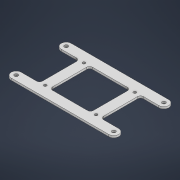
# Autodesk Inventor part: Mount Base
Saved by Autodesk Inventor 2021 (Build 250183000, 183)
## iProperties
Created: 2025-01-15
Part Number: Mount Base
Material: Generic
Document SubType Name: Modeling
Designer: user
Density: 1 g/cm^3
Appearance: Default
Author: user
Autodesk Inventor part; units mm, degrees
ref_plane "YZ Plane" through (0, 0, 0) normal (1, 0, 0) x (0, 1, 0)
ref_plane "XZ Plane" through (0, 0, 0) normal (0, 1, 0) x (-1, 0, 0)
ref_plane "XY Plane" through (0, 0, 0) normal (0, 0, 1) x (1, 0, 0)
sketch "Sketch1" plane through (0, 0, 0) normal (0, 1, 0) x (-1, 0, 0)
  line L0 (-7, 37.9777) -> (-7, 79.4722)
  spline S0 degree 3 poles (-7, 79.4722) (-7, 80.2679) (-6.8804, 81.313) (-5.8043, 84.1015) (-4.8936, 85.3942) (-3.1709, 87.6073) (-2.4028, 88.4658) (-2.0131, 89.2627) (-1.9647, 89.4035) (-1.9309, 89.6007) (-1.9254, 89.6626) (-1.9254, 89.7249) knots 0 0 0 0 0.238712 0.238712 0.524177 0.524177 0.81278 0.81278 0.88277 0.88277 0.915008 0.915008 0.915008 0.915008
  line L1 (0, 89.7249) -> (-1.9254, 89.7249)
  line L2 (0, 111.4478) -> (0, 89.7249)
  arc A0 (-6.2149, 117.4498) -> (0, 111.4478) centre (-2.5273, 115.0495) ccw
  line L3 (-135.9053, 117.4498) -> (-6.2149, 117.4498)
  arc A1 (-141.8339, 111.5213) -> (-135.9053, 117.4498) centre (-139.8146, 115.4305) ccw
  line L4 (-141.8339, 89.7249) -> (-141.8339, 111.5213)
  line L5 (-139.9085, 89.7249) -> (-141.8339, 89.7249)
  spline S1 degree 3 poles (-134.8339, 79.4722) (-134.8339, 80.1182) (-134.9165, 80.7597) (-135.2383, 82.0916) (-135.4922, 82.7684) (-136.3337, 84.5039) (-137.0038, 85.4638) (-138.2583, 87.0963) (-138.8405, 87.7821) (-139.5233, 88.7046) (-139.7055, 88.9932) (-139.8538, 89.363) (-139.888, 89.4816) (-139.9062, 89.645) (-139.9085, 89.685) (-139.9085, 89.7249) knots -1.843204 -1.843204 -1.843204 -1.843204 -1.717345 -1.717345 -1.576636 -1.576636 -1.342905 -1.342905 -1.132569 -1.132569 -0.995579 -0.995579 -0.934295 -0.934295 -0.914246 -0.914246 -0.914246 -0.914246
  line L6 (-134.8339, 79.4722) -> (-134.8339, 37.9777)
  spline S2 degree 3 poles (-134.8339, 37.9777) (-134.8339, 37.182) (-134.9535, 36.1368) (-136.0296, 33.3484) (-136.9403, 32.0557) (-138.663, 29.8425) (-139.4311, 28.984) (-139.8208, 28.1872) (-139.8692, 28.0464) (-139.903, 27.8492) (-139.9085, 27.7873) (-139.9085, 27.7249) knots 0 0 0 0 0.238712 0.238712 0.524177 0.524177 0.81278 0.81278 0.88277 0.88277 0.915008 0.915008 0.915008 0.915008
  line L7 (-141.8339, 27.7249) -> (-139.9085, 27.7249)
  line L8 (-141.8339, 5.9286) -> (-141.8339, 27.7249)
  arc A2 (-135.9053, 0) -> (-141.8339, 5.9286) centre (-139.8146, 2.0193) ccw
  line L9 (-6.0879, 0) -> (-135.9053, 0)
  arc A3 (0, 6.0879) -> (-6.0879, 0) centre (-2.4003, 2.4003) ccw
  line L10 (0, 27.7249) -> (0, 6.0879)
  line L11 (-1.9254, 27.7249) -> (0, 27.7249)
  spline S3 degree 3 poles (-7, 37.9777) (-7, 37.3317) (-6.9174, 36.6902) (-6.5955, 35.3583) (-6.3417, 34.6814) (-5.5001, 32.9459) (-4.8301, 31.986) (-3.5755, 30.3535) (-2.9934, 29.6677) (-2.3106, 28.7453) (-2.1284, 28.4567) (-1.9801, 28.0868) (-1.9459, 27.9682) (-1.9277, 27.8049) (-1.9254, 27.7649) (-1.9254, 27.7249) knots -1.843204 -1.843204 -1.843204 -1.843204 -1.717345 -1.717345 -1.576636 -1.576636 -1.342905 -1.342905 -1.132569 -1.132569 -0.995579 -0.995579 -0.934295 -0.934295 -0.914246 -0.914246 -0.914246 -0.914246
  circle A4 centre (-121.8339, 20) radius 2.75
  line L12 (-121.8339, 24.7343) -> (-117.7339, 22.3671)
  line L13 (-117.7339, 22.3671) -> (-117.7339, 17.6329)
  line L14 (-117.7339, 17.6329) -> (-121.8339, 15.2657)
  line L15 (-121.8339, 15.2657) -> (-125.9339, 17.6329)
  line L16 (-125.9339, 17.6329) -> (-125.9339, 22.3671)
  line L17 (-125.9339, 22.3671) -> (-121.8339, 24.7343)
  line L18 (-134.8339, 39.0386) -> (-134.8339, 78.4112)
  line L19 (-134.8339, 58.7249) -> (-125.9339, 58.7249)
  line L20 (-70.9966, 0) -> (-70.9966, 6.0879)
  line L21 (-117.7339, 95.0827) -> (-117.7339, 99.817)
  line L22 (-117.7339, 99.817) -> (-121.8339, 102.1841)
  line L23 (-125.9339, 95.0827) -> (-121.8339, 92.7156)
  line L24 (-125.9339, 99.817) -> (-125.9339, 95.0827)
  circle A5 centre (-121.8339, 97.4498) radius 2.75
  line L25 (-121.8339, 102.1841) -> (-125.9339, 99.817)
  line L26 (-121.8339, 92.7156) -> (-117.7339, 95.0827)
  line L27 (-24.2593, 22.3671) -> (-24.2593, 17.6329)
  line L28 (-20.1593, 24.7343) -> (-24.2593, 22.3671)
  line L29 (-24.2593, 17.6329) -> (-20.1593, 15.2657)
  circle A6 centre (-20.1593, 20) radius 2.75
  line L30 (-16.0593, 17.6329) -> (-16.0593, 22.3671)
  line L31 (-20.1593, 15.2657) -> (-16.0593, 17.6329)
  line L32 (-16.0593, 22.3671) -> (-20.1593, 24.7343)
  line L33 (-20.1593, 92.7156) -> (-24.2593, 95.0827)
  line L34 (-24.2593, 95.0827) -> (-24.2593, 99.817)
  line L35 (-16.0593, 99.817) -> (-16.0593, 95.0827)
  circle A7 centre (-20.1593, 97.4498) radius 2.75
  line L36 (-24.2593, 99.817) -> (-20.1593, 102.1841)
  line L37 (-20.1593, 102.1841) -> (-16.0593, 99.817)
  line L38 (-16.0593, 95.0827) -> (-20.1593, 92.7156)
  circle A8 centre (-121.8339, 20) radius 7.5
  circle A9 centre (-121.8339, 97.4498) radius 7.5
  circle A10 centre (-20.1593, 20) radius 7.5
  circle A11 centre (-20.1593, 97.4498) radius 7.5
  line L39 (26.5034, 108.7249) -> (-168.4966, 108.7249) construction
  line L40 (26.5034, 118.7249) -> (-168.4966, 118.7249)
  line L41 (-168.4966, 98.7249) -> (26.5034, 98.7249)
  arc A12 (26.5034, 98.7249) -> (26.5034, 118.7249) centre (26.5034, 108.7249) ccw
  arc A13 (-168.4966, 118.7249) -> (-168.4966, 98.7249) centre (-168.4966, 108.7249) ccw
  circle A14 centre (26.5034, 108.7249) radius 3.6
  circle A15 centre (-168.4966, 108.7249) radius 3.6
  line L42 (-121.8339, 97.4498) -> (-20.1593, 97.4498)
  line L43 (-20.1593, 97.4498) -> (-20.1593, 20)
  line L44 (26.5034, 8.7249) -> (26.5034, 108.7249)
  line L45 (-168.4966, 108.7249) -> (-168.4966, 8.7249)
  line L46 (26.5034, 8.7249) -> (-168.4966, 8.7249) construction
  line L47 (26.5034, 18.7249) -> (-168.4966, 18.7249)
  line L48 (-168.4966, -1.2751) -> (26.5034, -1.2751)
  arc A16 (26.5034, -1.2751) -> (26.5034, 18.7249) centre (26.5034, 8.7249) ccw
  arc A17 (-168.4966, 18.7249) -> (-168.4966, -1.2751) centre (-168.4966, 8.7249) ccw
  circle A18 centre (26.5034, 8.7249) radius 3.6
  circle A19 centre (-168.4966, 8.7249) radius 3.6
  line L49 (-20.1593, 20) -> (-20.1593, 97.4498) construction
  line L50 (-10.1593, 18.7249) -> (-10.1593, 98.7249)
  line L51 (-30.1593, 98.7249) -> (-30.1593, 18.7249)
  line L52 (-121.8339, 20) -> (-121.8339, 97.4498) construction
  line L53 (-111.8339, 18.7249) -> (-111.8339, 98.7249)
  line L54 (-131.8339, 98.7249) -> (-131.8339, 18.7249)
  point P0 (0, 0)
  point P1 (0, 0)
  point P2 (-16.0593, 58.7249)
  point P3 (-70.9966, 108.7249)
  point P4 (-70.9966, 97.4498)
  point P5 (26.5034, 58.7249)
  point P6 (-20.1593, 58.7249)
  point P7 (-70.9966, 8.7249)
  point P8 (-20.1593, 58.7249)
  point P9 (-121.8339, 58.7249)
  dimension "d0" = 5.5
  dimension "d1" = 8.2
  dimension "d2" = 20
  dimension "d3" = 20
  dimension "d4" = 15
  dimension "d5" = 195
  dimension "d6" = 20
  dimension "d7" = 7.2
  dimension "d8" = 7.2
  dimension "d9" = 100
  dimension "d10" = 20
  dimension "d11" = 7.2
  dimension "d12" = 7.2
  constraints: 118 end point, 28 symmetric about line, 20 centre point, 16 point on circle, 9 coincident, 9 midpoint, 8 point on line, 8 tangent, 5 parallel, 3 perpendicular, 3 vertical, 2 horizontal, 1 collinear, 1 horizontal alignment, 30 other
  measures "d0" diameter of A4
  measures "d1" distance between parallel lines of L13 L16
  measures "d2" distance from line of L8 A4.centre
  measures "d3" distance from line of L9 A4.centre
  measures "d4" diameter of A8
  measures "d5" distance of L39.start L39.end
  measures "d6" diameter of A13
  measures "d7" diameter of A14
  measures "d8" diameter of A15
  measures "d9" distance of L44.start L44.end
  measures "d10" diameter of A17
  measures "d11" diameter of A18
  measures "d12" diameter of A19
extrude "Extrusion1" add sketch "Sketch1" along normal blind 4 contours L47 A16 L48 A17 L8 A2 L9 A3 L10 | L10 A3 L9 A2 L8 L47 A8 A10 | L41 A11 A9 L4 A1 L3 A0 L2 | L2 A0 L3 A1 L4 L41 A13 L40 A12 | L47 A10 L43 A11 L41 L50 | L47 L30 L32 L43 A10 | A10 L47 L27 L29 L31 L30 | L41 L35 L37 L36 L34 A11 | A11 L43 L38 L35 L41 | L47 L51 L42 A11 L43 A10 | A10 L43 L28 L27 L47 | L47 A6 L43 L32 L30 | L30 L31 L29 L27 L47 A6 | L41 L34 L42 A11 | A11 L42 L51 L41 | L41 A7 L34 L36 L37 L35 | L35 L38 L43 A7 L41 | L27 L28 L43 A6 L47 | A11 L42 L34 L33 L43 | L41 A7 L42 L34 | L47 A8 L54 L41 A9 L42 L53 | L33 L34 L42 A7 L43 | L53 L42 A9 L41 | L47 L13 L12 L17 L16 A8 | A8 L47 L16 L15 L14 L13 | L41 L21 L22 L25 L24 A9 | A9 L42 L21 L41 | L47 A4 L16 L17 L12 L13 | L13 L14 L15 L16 L47 A4 | A9 L41 L24 L23 L26 L21 L42 | L41 A5 L24 L25 L22 L21 | L21 L42 A5 L41 | L21 L26 L23 L24 L41 A5 L42
fillet "Fillet1" radius 6 8 edges at (30.1593, 2, 98.7249) (10.1593, 2, 98.7249) (10.1593, 2, 18.7249) (30.1593, 2, 18.7249) (111.8339, 2, 18.7249) (131.8339, 2, 18.7249) (111.8339, 2, 98.7249) (131.8339, 2, 98.7249)
body "Solid1"
